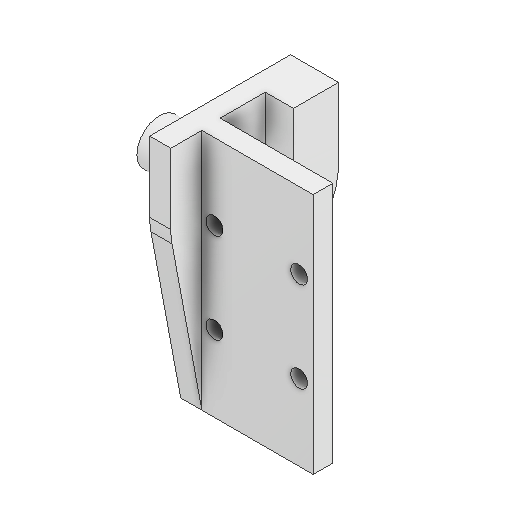
# Autodesk Inventor part: CarriagePivotMountMirror
Saved by Autodesk Inventor 2026.2 (Build 302298000, 298)
## iProperties
Created: 2026-03-23
Part Number: CarriagePivotMountMirror
Material: ABS Plastic
Document SubType Name: Modeling
Designer: gaoet
Density: 1.06 g/cm^3
Appearance: Smooth - White
Author: gaoet
Autodesk Inventor part; units mm, degrees
ref_plane "YZ Plane" through (0, 0, 0) normal (1, 0, 0) x (0, 1, 0)
ref_plane "XZ Plane" through (0, 0, 0) normal (0, 1, 0) x (-1, 0, 0)
sketch "Sketch1" plane through (0, 0, 0) normal (0, 0, 1) x (1, 0, 0)
  line L0 (-10, -21.5) -> (10, -21.5)
  line L1 (10, -21.5) -> (10, 21.5)
  line L2 (10, 21.5) -> (-10, 21.5)
  line L3 (-10, 21.5) -> (-10, -21.5)
  line L4 (-10, -21.5) -> (10, 21.5) construction
  line L5 (10, -21.5) -> (-10, 21.5) construction
  point P0 (0, 0)
  dimension "d0" = 20
  dimension "d1" = 43
  constraints: 12 end point, 2 midpoint, 2 parallel, 1 horizontal, 1 perpendicular
  measures "d0" distance of L2.end L1.end
  measures "d1" distance of L1.end L0.end
extrude "Extrusion1" add sketch "Sketch1" along normal blind 3.5
sketch "Sketch2" plane through (0, 0, 3.5) normal (0, 0, 1) x (1, 0, 0)
  line L0 (-7.5, -8) -> (7.5, -8)
  line L1 (7.5, -8) -> (7.5, 8)
  line L2 (7.5, 8) -> (-7.5, 8)
  line L3 (-7.5, 8) -> (-7.5, -8)
  line L4 (-7.5, -8) -> (7.5, 8) construction
  line L5 (7.5, -8) -> (-7.5, 8) construction
  point P0 (0, 0)
  dimension "d4" = 15
  dimension "d5" = 16
  constraints: 12 end point, 2 midpoint, 2 parallel, 1 horizontal, 1 perpendicular
  measures "d4" distance of L2.end L1.end
  measures "d5" distance of L1.end L0.end
hole "Hole1" at (-7.5, 8, 3.5) at (7.5, 8, 3.5) at (7.5, -8, 3.5) at (-7.5, -8, 3.5) direction (0, 0, -1) diameter 3 end through all
sketch "Sketch3" plane through (10, -21.5, 0) normal (1, 0, 0) x (0, 0, -1)
  circle A0 centre (3.5, 30.5) radius 11.9062
  line L0 (0, 0) -> (0, 43) projected
  circle A1 centre (3.5, 30.5) radius 12.5
  line L1 (0, 43) -> (3.5, 43)
  line L2 (14.2623, 24.142) -> (0, 0)
  line L3 (-3.5, 43) -> (-3.5, 0) projected
  line L4 (-3.5, 43) -> (-7.1577, 37.0317)
  line L5 (-3.5, 0) -> (-8.786, 28.1968)
  line L6 (0, 0) -> (-3.5, 0) projected
  line L7 (0, 43) -> (-3.5, 43) projected
  line L8 (16, 30.5) -> (16, 43)
  line L9 (16, 43) -> (-9, 43)
  line L10 (-9, 43) -> (-9, 30.5)
  line L11 (9, 43) -> (12.7158, 38.945)
  point P0 (0, 21.5)
  point P1 (0, 21.5)
  point P2 (3.5, 43)
  dimension "d14" = 25
  dimension "d13" = 23.8125
  dimension "d15" = 3.5
  dimension "d26" = 9
  constraints: 16 end point, 4 vertical, 2 horizontal, 1 centre point, 1 coincident, 1 collinear, 1 midpoint, 1 perpendicular, 1 point on line, 13 other
  measures "d13" diameter of A0
  measures "d15" distance from line of L0 A0.centre
  measures "d26" distance of L0.end L11.start
extrude "Extrusion2" add sketch "Sketch3" along normal blind 3.5
sketch "Sketch4" plane through (13.5, -21.5, 0) normal (1, 0, 0) x (0, 0, -1)
  circle A0 centre (3.5, 30.5) radius 11.9062 projected
  point P0 (0, 21.5)
extrude "Extrusion3" add sketch "Sketch4" along normal blind 0.5
sketch "Sketch5" plane through (10, -21.5, 0) normal (-1, 0, 0) x (0, 0, 1)
  line L0 (3.5, 0) -> (3.5, 43) projected
  line L1 (8.786, 28.1968) -> (3.5, 0) projected
  arc A0 (-16, 30.5) -> (-14.2623, 24.142) centre (-3.5, 30.5) ccw projected
  arc A1 (8.786, 28.1968) -> (9, 30.5) centre (-3.5, 30.5) ccw projected
  line L2 (0, 0) -> (0, 43) projected
  line L3 (0, 0) -> (-14.2623, 24.142) projected
  line L4 (-16, 43) -> (0, 43) projected
  line L5 (-16, 30.5) -> (-16, 43) projected
  line L6 (9, 43) -> (9, 30.5) projected
  line L7 (3.5, 43) -> (9, 43) projected
  point P0 (0, 21.5)
extrude "Extrusion4" add sketch "Sketch5" along normal blind 0.25
sketch "Sketch6" plane through (10, -21.5, 0) normal (-1, 0, 0) x (0, 0, 1)
  line L0 (-14.2623, 24.142) -> (0, 0) projected
  line L1 (0, 43) -> (0, 0) projected
  line L2 (0, 43) -> (-16, 43) projected
  line L3 (-16, 43) -> (-16, 30.5) projected
  arc A0 (-16, 30.5) -> (-14.2623, 24.142) centre (-3.5, 30.5) ccw projected
  line L4 (-8, 13.5418) -> (-8, 43)
  dimension "d67" = 8
  constraints: 2 end point, 1 midpoint, 1 perpendicular, 1 point on line
  measures "d67" distance between parallel lines of L1 L4
extrude "Extrusion5" add sketch "Sketch6" along normal blind 5 contours A0 L3 L2 L4 L0
sketch "Sketch7" plane through (14, 9, -3.5) normal (1, 0, 0) x (0, 0, -1)
  circle A0 centre (0, 0) radius 11.9062 projected
  circle A1 centre (0, 0) radius 6.1
  circle A2 centre (-2, 3.4641) radius 1.5
  circle A3 centre (4, 0) radius 1.5
  circle A4 centre (-2, -3.4641) radius 1.5
  line L0 (-2, 3.4641) -> (0, 0) construction
  line L1 (0, 0) -> (4, 0) construction
  line L2 (-2, -3.4641) -> (0, 0) construction
  circle A5 centre (0, 0) radius 2
  point P0 (-3.5, -9)
  dimension "d27" = 12.2
  dimension "d28" = 3
  dimension "d29" = 120
  dimension "d30" = 120
  dimension "d31" = 4
  dimension "d32" = 4
  constraints: 6 end point, 5 centre point, 2 coincident, 2 equal length, 2 equal radius, 1 horizontal
  measures "d27" diameter of A1
  measures "d28" diameter of A2
  measures "d29" angle of L1 L0
  measures "d30" angle of L2 L0
  measures "d31" distance of L0.start L0.end
  measures "d32" diameter of A5
sketch "Sketch10" plane through (14, 9, -3.5) normal (1, 0, 0) x (0, 0, -1)
  circle A0 centre (0, 0) radius 11.9062 projected
  circle A1 centre (0, 0) radius 6.1
  point P0 (-3.5, -9)
  dimension "d44" = 12.2
  constraints: 1 centre point, 1 coincident
  measures "d44" diameter of A1
extrude "Extrusion7" add sketch "Sketch10" along normal blind 5.28 contours A1
sketch "Sketch11" plane through (19.28, 9, -3.5) normal (1, 0, 0) x (0, 0, -1)
  circle A0 centre (0, 0) radius 6.1 projected
  circle A1 centre (0, 0) radius 4
  point P0 (-3.5, -9)
  dimension "d47" = 8
  constraints: 1 centre point, 1 coincident
  measures "d47" diameter of A1
extrude "Extrusion8" add sketch "Sketch11" along normal blind 5 contours A1
sketch "Sketch12" plane through (24.28, 9, -3.5) normal (1, 0, 0) x (0, 0, -1)
  circle A0 centre (0, 0) radius 4 projected
  point P0 (-3.5, -9)
hole "Hole3" at (24.28, 9, -3.5) direction (-1, 0, 0) diameter 4 end through all
sketch "Sketch13" plane through (10, -21.5, 0) normal (-1, 0, 0) x (0, 0, 1)
  circle A0 centre (-3.5, 30.5) radius 2 projected
  line L0 (-8, 43) -> (-8, 13.5418) projected
  line L1 (-8, 13.5418) -> (0, 0) projected
  line L2 (0, 43) -> (0, 0) projected
  line L3 (0, 43) -> (-8, 43) projected
  line L4 (-7, 32.5207) -> (-3.5, 34.5415)
  line L5 (-3.5, 34.5415) -> (0, 32.5207)
  line L6 (0, 32.5207) -> (0, 28.4793)
  line L7 (0, 28.4793) -> (-3.5, 26.4585)
  line L8 (-3.5, 26.4585) -> (-7, 28.4793)
  line L9 (-7, 28.4793) -> (-7, 32.5207)
  point P0 (-7, 30.5)
  point P1 (0, 28.4793)
  point P2 (0, 32.5207)
  dimension "d68" = 7
  constraints: 12 end point, 1 coincident, 1 midpoint, 1 vertical, 13 other
  measures "d68" distance from line of L6 point (-7, 30.5)
extrude "Extrusion9" cut sketch "Sketch13" against normal blind 3.7 contours L2 L7 L8 L9 L4 L5
sketch "Sketch15" plane through (19.28, 9, -3.5) normal (1, 0, 0) x (0, 0, -1)
  circle A0 centre (0, 0) radius 4 projected
  circle A1 centre (0, 0) radius 6.1 projected
  line L0 (3.75, 4.8112) -> (-3.75, 4.8112)
  point P0 (-3.5, -9)
  dimension "d62" = 7.5
  constraints: 2 end point, 2 point on circle, 1 horizontal
  measures "d62" distance of L0.start L0.end
extrude "Extrusion11" cut sketch "Sketch15" against normal up to surface (5.28 mm away) contours L0 A1 picked at (-0.8686, 5.0459)
sketch "Sketch17" plane through (9.75, -21.5, 0) normal (-1, 0, 0) x (0, 0, 1)
  line L0 (-7, 28.4793) -> (-7, 32.5207) projected
  line L1 (-3.5, 26.4585) -> (-7, 28.4793) projected
  line L2 (0, 28.4793) -> (-3.5, 26.4585) projected
  line L3 (0, 32.5207) -> (0, 28.4793) projected
  line L4 (-3.5, 34.5415) -> (0, 32.5207) projected
  line L5 (-7, 32.5207) -> (-3.5, 34.5415) projected
  circle A0 centre (-3.5, 30.5) radius 2 projected
  point P0 (0, 21.5)
extrude "Extrusion13" cut sketch "Sketch17" against normal blind 3.7 contours L0 L5 L4 L3 L2 L1 | A0
fillet "Fillet2" radius 1 1 edges at (7.375, -7.9582, -8)
sketch "Sketch18" plane through (9.75, -21.5, 0) normal (-1, 0, 0) x (0, 0, 1)
  line L0 (0, 28.4793) -> (-3.5, 26.4585) projected
  line L1 (-3.5, 26.4585) -> (-7, 28.4793) projected
  line L2 (-7, 28.4793) -> (-7, 32.5207) projected
  line L3 (-7, 32.5207) -> (-3.5, 34.5415) projected
  line L4 (-3.5, 34.5415) -> (0, 32.5207) projected
  line L5 (0, 43) -> (0, 32.5207) projected
  line L6 (0, 43) -> (-8, 43) projected
  line L7 (-8, 43) -> (-8, 17.2005) projected
  arc A0 (-9.861, 16.6919) -> (-8, 17.2005) centre (-9, 17.2005) ccw projected
  line L8 (-9.861, 16.6919) -> (0, 0) projected
  line L9 (0, 28.4793) -> (0, 0) projected
  point P0 (0, 21.5)
extrude "Extrusion14" cut sketch "Sketch18" against normal blind 0.25
ref_plane "Work Plane1" through (-11, -21.5, 0) normal (-1, 0, 0) x (0, 0, 1)
mirror "Mirror1" about plane through (-11, -21.5, 0) normal (-1, 0, 0) of "Extrusion1", "Hole1", "Extrusion2", "Extrusion3", "Extrusion4", "Extrusion5", "Extrusion7", "Extrusion8", "Hole3", "Extrusion9", "Extrusion11", "Extrusion13", "Fillet2", "Extrusion14"
sketch "Sketch19" plane through (-11, -21.5, 0) normal (-1, 0, 0) x (0, 0, 1)
  line L0 (-26.4701, -15.0074) -> (17.4098, -15.0074)
  line L1 (17.4098, -15.0074) -> (17.4098, 56.4974)
  line L2 (17.4098, 56.4974) -> (-26.4701, 56.4974)
  line L3 (-26.4701, 56.4974) -> (-26.4701, -15.0074)
  point P0 (0, 21.5)
  constraints: 8 end point, 2 parallel, 1 horizontal, 1 perpendicular
extrude "Extrusion15" cut sketch "Sketch19" against normal through all
equation "\"d30\" = d29"
body "Solid1"
